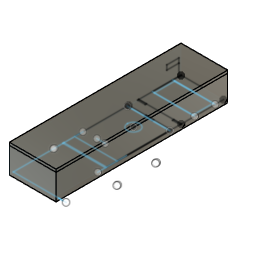
remotecase (Autodesk Fusion 360 design; units mm, degrees)
Autodesk Fusion 360 part; units mm, degrees
sketch "Sketch1" plane through (0, 0, 0) normal (0, 0, 1) x (1, 0, 0)
  line L0 (0, 0) -> (31, 0)
  line L1 (31, 0) -> (31, 114)
  line L2 (31, 114) -> (0, 114)
  line L3 (0, 114) -> (0, 0)
  dimension "d1" = 31
  dimension "d2" = 114
  constraint horizontal L0
  constraint vertical L1
  constraint horizontal L2
  constraint vertical L3
  constraint coincident L0.start L3.end
  measures "d1" distance of L0.start L0.end
  measures "d2" distance of L0.start L2.end
extrude "Extrude1" add sketch "Sketch1" along normal blind 9 makes body 1
sketch "Sketch2" plane through (0, 0, 9) normal (0, 0, 1) x (-1, 0, 0)
  line L0 (0, -114) -> (0, 0)
  line L1 (0, 0) -> (-31, 0)
  line L2 (-31, 0) -> (-31, -114)
  line L3 (-31, -114) -> (0, -114)
  line L4 (0, 0) -> (-1.4, 0)
  line L5 (-1.4, 0) -> (-1.4, -1.4)
  line L6 (-31, -114) -> (-29.6, -114)
  line L7 (-29.6, -114) -> (-29.6, -112.6)
  line L8 (-1.4, -1.4) -> (-29.6, -1.4)
  line L9 (-29.6, -1.4) -> (-29.6, -112.6)
  line L10 (-29.6, -112.6) -> (-1.4, -112.6)
  line L11 (-1.4, -112.6) -> (-1.4, -1.4)
  dimension "d5" = 1.4
  dimension "d6" = 1.4
  dimension "d7" = 1.4
  dimension "d8" = 1.4
  constraint coincident L0.end L1.start
  constraint perpendicular L0 L4
  constraint perpendicular L1 L5
  constraint coincident L2.end L3.start
  constraint perpendicular L2 L6
  constraint perpendicular L6 L7
  constraint horizontal L8
  constraint vertical L9
  constraint horizontal L10
  constraint vertical L11
  measures "d5" distance of L0.end L4.end
  measures "d6" distance of L4.end L5.end
  measures "d7" distance of L2.end L6.end
  measures "d8" distance of L6.end L7.end
extrude "Extrude2" cut sketch "Sketch2" against normal blind 7.2 contours L8 L9 L10 L11 bodies 1
sketch "Sketch3" plane through (0, 0, 1.8) normal (0, 0, 1) x (-1, 0, 0)
  line L0 (-1.4, -112.6) -> (-1.4, -1.4)
  line L1 (-1.4, -1.4) -> (-29.6, -1.4)
  line L2 (-29.6, -1.4) -> (-29.6, -112.6)
  line L3 (-29.6, -112.6) -> (-1.4, -112.6)
  line L4 (-29.6, -76.9421) -> (-29.6, -48.1421)
  line L5 (-15.5, -48.1421) -> (-10, -48.1421)
  line L6 (-1.4, -76.9421) -> (-29.6, -76.9421)
  line L7 (-15.5, -112.6) -> (-1.5, -112.6)
  line L8 (-1.5, -107.1) -> (-1.5, -112.6)
  line L9 (-1.5, -93.6) -> (-1.5, -107.1)
  line L10 (-29.6, -48.1421) -> (-29.6, -29.1421)
  line L11 (-43.6, -54.1421) -> (-43.6, -53.4421)
  line L12 (-1.4, -28.4421) -> (-1.4, -47.4421)
  line L13 (-43.6, -28.4421) -> (-43.6, -27.7421)
  line L14 (-36.4, -1.2421) -> (-1.4, -1.2421)
  line L15 (-1.4, -1.2421) -> (-1.4, -27.7421)
  line L16 (-15.5, -76.9421) -> (-15.5, -66.9421)
  circle A0 centre (-15.5, -66.9421) radius 4
  line L17 (-29.6, -76.9421) -> (-29.6, -41.9421)
  line L18 (-29.6, -41.9421) -> (-1.4, -41.9421)
  line L19 (-1.4, -41.9421) -> (-1.4, -76.9421)
  line L20 (-1.4, -76.9421) -> (-29.6, -76.9421)
  line L21 (-29.6, -76.9421) -> (-29.6, -41.9421)
  line L22 (-29.6, -41.9421) -> (-29.6, -34.9421)
  line L23 (-29.6, -34.9421) -> (-1.4, -34.9421)
  line L24 (-1.4, -34.9421) -> (-1.4, -34.2421)
  line L25 (-1.4, -34.2421) -> (-29.6, -34.2421)
  line L26 (-29.6, -34.2421) -> (-29.6, -34.9421)
  line L27 (-1.5, -107.1) -> (-29.5, -107.1074)
  line L28 (-1.5, -93.6) -> (-29.5, -93.5275)
  line L29 (-15.5, -107.1037) -> (-2.75, -107.1003)
  line L30 (-2.75, -107.1003) -> (-28.25, -107.1003)
  line L31 (-28.25, -107.1003) -> (-28.25, -93.5638)
  line L32 (-28.25, -93.5638) -> (-2.75, -93.5638)
  line L33 (-2.75, -93.5638) -> (-2.75, -107.1003)
  line L34 (-1.4, -112.6) -> (-1.4, -84.6)
  line L35 (-1.4, -84.6) -> (-6.4, -84.6)
  line L36 (-6.4, -84.6) -> (-6.4, -83.8)
  line L37 (-6.4, -83.8) -> (-1.4, -83.8)
  line L38 (-1.4, -83.8) -> (-1.4, -84.6)
  line L39 (-1.4, -84.6) -> (-29.6, -84.6)
  line L40 (-29.6, -84.6) -> (-24.6, -84.6)
  line L41 (-24.6, -84.6) -> (-24.6, -83.8)
  line L42 (-24.6, -83.8) -> (-29.6, -83.8)
  line L43 (-29.6, -83.8) -> (-29.6, -84.6)
  line L44 (-29.6, -112.6) -> (-29.6, -77.8)
  line L45 (-29.6, -77.8) -> (-1.4, -77.8)
  line L46 (-15.5, -77.8) -> (-13, -77.8)
  line L47 (-13, -77.8) -> (-18, -77.8)
  line L48 (-18, -77.8) -> (-18, -77)
  line L49 (-18, -77) -> (-13, -77)
  line L50 (-13, -77) -> (-13, -77.8)
  dimension "d23" = 14
  dimension "d25" = 5.5
  dimension "d26" = 13.5
  dimension "d53" = 10
  dimension "d54" = 8
  dimension "d58" = 35
  dimension "d59" = 7
  dimension "d60" = 0.7
  dimension "d61" = 12.75
  dimension "d62" = 25.5
  dimension "d122" = 28
  dimension "d123" = 5
  dimension "d124" = 0.8
  dimension "d125" = 5
  dimension "d126" = 0.8
  dimension "d131" = 34.8
  dimension "d132" = 2.5
  dimension "d133" = 5
  dimension "d134" = 0.8
  constraint coincident L2 L4.start
  constraint parallel L2 L4
  constraint perpendicular L0 L5
  constraint coincident L0 L6.start
  constraint perpendicular L4 L6
  constraint midpoint L3 L7.start
  constraint perpendicular L0 L7
  constraint vertical L8
  constraint vertical L9
  constraint vertical L11
  constraint vertical L12
  constraint vertical L13
  constraint horizontal L14
  constraint vertical L15
  constraint midpoint L6 L16.start
  constraint perpendicular L6 L16
  constraint coincident L16.end A0.centre
  constraint perpendicular L6 L17
  constraint horizontal L18
  constraint vertical L19
  constraint horizontal L20
  constraint vertical L21
  constraint perpendicular L18 L22
  constraint horizontal L23
  constraint vertical L24
  constraint horizontal L25
  constraint vertical L26
  constraint midpoint L27 L29.start
  constraint parallel L27 L29
  constraint horizontal L30
  constraint vertical L31
  constraint horizontal L32
  constraint vertical L33
  constraint coincident L0.start L3.end
  constraint perpendicular L3 L34
  constraint horizontal L35
  constraint vertical L36
  constraint horizontal L37
  constraint vertical L38
  constraint horizontal L39
  constraint coincident L2 L39.end
  constraint horizontal L40
  constraint vertical L41
  constraint horizontal L42
  constraint vertical L43
  constraint coincident L2.end L3.start
  constraint perpendicular L32 L44
  constraint coincident L0 L45.end
  constraint perpendicular L0 L45
  constraint midpoint L45 L46.start
  constraint parallel L45 L46
  constraint horizontal L47
  constraint vertical L48
  constraint horizontal L49
  constraint vertical L50
  measures "d23" distance of L7.start L7.end
  measures "d25" distance of L7.end L8.start
  measures "d26" distance of L8.start L9.start
  measures "d53" distance of L16.start L16.end
  measures "d54" diameter of A0
  measures "d58" distance of L4.start L17.end
  measures "d59" distance of L17.end L22.end
  measures "d60" distance of L22.end L25.end
  measures "d61" distance of L29.start L29.end
  measures "d62" distance of L29.end L30.end
  measures "d122" distance of L0.start L34.end
  measures "d123" distance of L34.end L35.end
  measures "d124" distance of L34.end L37.end
  measures "d125" distance of L39.end L40.end
  measures "d126" distance of L39.end L42.end
  measures "d131" distance of L2.end L44.end
  measures "d132" distance of L46.start L46.end
  measures "d133" distance of L46.end L47.end
  measures "d134" distance of L46.end L49.end
extrude "Extrude10" cut sketch "Sketch3" against normal blind 6 contours L28 L30 L31 L32 L33 bodies 1
extrude "Extrude11" cut sketch "Sketch3" against normal blind 6 contours A0 bodies 1
extrude "Extrude12" add 1 faces at (30.5333, 38.4667, 9) along direction (0, 0, 1) blind 8 on bodies 1 bodies 1
sketch "Sketch8" plane through (0, 114, 0) normal (0, 1, 0) x (-1, 0, 0)
  line L0 (-31, 0) -> (0, 0)
  line L1 (0, 0) -> (0, 17)
  line L2 (0, 17) -> (-31, 17)
  line L3 (-31, 17) -> (-31, 0)
  line L4 (-15.5, 0) -> (-15.5, 8)
  line L5 (-15.5, 8) -> (-27.5, 8)
  line L6 (-27.5, 8) -> (-27.5, 15)
  line L7 (-27.5, 15) -> (-15.5, 15)
  line L8 (-15.5, 15) -> (-15.5, 8)
  dimension "d74" = 8
  dimension "d75" = 12
  dimension "d76" = 7
  constraint midpoint L0 L4.start
  constraint perpendicular L0 L4
  constraint horizontal L5
  constraint vertical L6
  constraint horizontal L7
  constraint vertical L8
  measures "d74" distance of L4.start L4.end
  measures "d75" distance of L4.end L5.end
  measures "d76" distance of L4.end L7.end
extrude "Extrude14" cut sketch "Sketch8" against normal blind 18 contours L5 L6 L7 L8 bodies 1
sketch "Sketch3 (2)" plane through (0, 0, 17) normal (0, 0, 1) x (-1, 0, 0) in component "kapak"
  line L0 (-29.6, -1.4) -> (-1.4, -1.4)
  line L1 (-1.4, -1.4) -> (-1.4, -112.6)
  line L2 (-1.4, -112.6) -> (-29.6, -112.6)
  line L3 (-29.6, -112.6) -> (-29.6, -1.4)
  line L4 (0, -114) -> (0, 0)
  line L5 (0, 0) -> (-31, 0)
  line L6 (-31, 0) -> (-31, -114)
  line L7 (-31, -114) -> (0, -114)
  line L8 (0, -114) -> (-31, -114)
  line L9 (-31, -114) -> (-31, 0)
  line L10 (-31, 0) -> (0, 0)
  line L11 (0, 0) -> (0, -114)
  constraint horizontal L8
  constraint vertical L9
  constraint horizontal L10
  constraint vertical L11
  constraint coincident L5.end L6.start
  constraint coincident L4.start L7.end
extrude "Extrude1'" add sketch "Sketch3 (2)" along normal blind 1.8 separate body contours L0 L1 L2 L3 | L4 L5 L6 L7 L8 L9 L10 L11 makes body 2 in component "kapak"
sketch "Sketch4" plane through (0, 0, 17) normal (0, 0, 1) x (1, 0, 0) in component "kapak"
  line L0 (1.4, 1.4) -> (29.6, 1.4)
  line L1 (29.6, 1.4) -> (29.6, 112.6)
  line L2 (29.6, 112.6) -> (1.4, 112.6)
  line L3 (1.4, 112.6) -> (1.4, 1.4)
  line L4 (1.4, 1.4) -> (2.8, 1.4)
  line L5 (1.4, 2.8) -> (1.4, 1.4)
  line L6 (29.6, 112.6) -> (28.2, 112.6)
  line L7 (29.6, 111.2) -> (29.6, 112.6)
  line L8 (28.2, 111.2) -> (2.8, 111.2)
  line L9 (2.8, 111.2) -> (2.8, 2.8)
  line L10 (2.8, 2.8) -> (28.2, 2.8)
  line L11 (28.2, 2.8) -> (28.2, 111.2)
  dimension "d90" = 1.4
  dimension "d91" = 1.4
  dimension "d92" = 1.4
  dimension "d93" = 1.4
  constraint horizontal L0
  constraint vertical L1
  constraint horizontal L2
  constraint vertical L3
  constraint horizontal L4
  constraint vertical L5
  constraint horizontal L8
  constraint vertical L9
  constraint horizontal L10
  constraint vertical L11
  measures "d90" distance of L0.start L4.end
  measures "d91" distance of L0.start L5.start
  measures "d92" distance of L1.end L6.end
  measures "d93" distance of L1.end L7.start
extrude "Extrude2'" add sketch "Sketch4" against normal blind 1.2 bodies 2 in component "kapak"
sketch "Sketch6" plane through (0, 0, 17) normal (0, 0, -1) x (1, 0, 0) in component "kapak"
  line L0 (31, 0) -> (0, 0)
  line L1 (0, 0) -> (0, -114)
  line L2 (0, -114) -> (31, -114)
  line L3 (31, -114) -> (31, 0)
  line L4 (29.6, -112.6) -> (1.4, -112.6)
  line L5 (1.4, -112.6) -> (1.4, -1.4)
  line L6 (1.4, -1.4) -> (29.6, -1.4)
  line L7 (29.6, -1.4) -> (29.6, -112.6)
  line L8 (15.5, -114) -> (15.5, -104)
  line L9 (15.5, -104) -> (15.1, -104)
  line L10 (15.1, -104) -> (15.9, -104)
  line L11 (15.9, -104) -> (15.9, -89)
  line L12 (15.9, -89) -> (15.1, -89)
  line L13 (15.1, -89) -> (15.1, -104)
  line L14 (15.5, -114) -> (15.5, -64)
  line L15 (15.5, -64) -> (15.1, -64)
  line L16 (15.1, -64) -> (16.5, -64)
  line L17 (16.5, -64) -> (16.5, -54)
  line L18 (16.5, -54) -> (15.1, -54)
  line L19 (15.1, -54) -> (15.1, -64)
  line L20 (15.5, 0) -> (15.5, -10)
  line L21 (15.5, -10) -> (15.1, -10)
  line L22 (15.1, -10) -> (15.9, -10)
  line L23 (15.9, -10) -> (15.9, -20)
  line L24 (15.9, -20) -> (15.1, -20)
  line L25 (15.1, -20) -> (15.1, -10)
  dimension "d96" = 10
  dimension "d97" = 0.4
  dimension "d98" = 0.8
  dimension "d99" = 15
  dimension "d100" = 50
  dimension "d101" = 0.4
  dimension "d102" = 1.4
  dimension "d103" = 10
  dimension "d104" = 10
  dimension "d105" = 0.4
  dimension "d106" = 0.8
  dimension "d107" = 10
  constraint midpoint L2 L8.start
  constraint perpendicular L2 L8
  constraint perpendicular L8 L9
  constraint horizontal L10
  constraint vertical L11
  constraint horizontal L12
  constraint vertical L13
  constraint vertical L14
  constraint perpendicular L14 L15
  constraint horizontal L16
  constraint vertical L17
  constraint horizontal L18
  constraint vertical L19
  constraint midpoint L0 L20.start
  constraint perpendicular L6 L20
  constraint perpendicular L20 L21
  constraint horizontal L22
  constraint vertical L23
  constraint horizontal L24
  constraint vertical L25
  measures "d96" distance of L8.start L8.end
  measures "d97" distance of L8.end L9.end
  measures "d98" distance of L9.end L10.end
  measures "d99" distance of L9.end L12.end
  measures "d100" distance of L8.start L14.end
  measures "d101" distance of L14.end L15.end
  measures "d102" distance of L15.end L16.end
  measures "d103" distance of L15.end L18.end
  measures "d104" distance of L20.start L20.end
  measures "d105" distance of L20.end L21.end
  measures "d106" distance of L21.end L22.end
  measures "d107" distance of L21.end L24.end
extrude "Extrude3" add sketch "Sketch6" along normal blind 7.5 contours L21 L22 L23 L24 L25 bodies 2 in component "kapak"
extrude "Extrude4" add sketch "Sketch6" along normal blind 8 contours L15 L16 L17 L18 L19 bodies 2 in component "kapak"
extrude "Extrude5" add sketch "Sketch6" along normal blind 3.5 contours L10 L11 L12 L14 | L9 L10 L12 L13 L14 bodies 2 in component "kapak"
extrude "Extrude6" add 1 faces at (16.0333, 60.6667, 9) along direction (0, 0, -1) blind 2 on bodies 2 bodies 2 in component "kapak"
sketch "Sketch9" plane through (0, 0, 0) normal (-1, 0, 0) x (0, -1, 0)
  line L0 (-114, 0) -> (0, 0)
  line L1 (0, 0) -> (0, 17)
  line L2 (0, 17) -> (-114, 17)
  line L3 (-114, 17) -> (-114, 0)
  line L4 (-114, 0) -> (-112.6, 0)
  line L5 (-112.6, 0) -> (-112.6, 8)
  line L6 (-112.6, 8) -> (-104.6, 8)
  line L7 (-104.6, 8) -> (-104.6, 11)
  line L8 (-104.6, 11) -> (-112.6, 11)
  line L9 (-112.6, 11) -> (-112.6, 8)
  dimension "d116" = 1.4
  dimension "d117" = 8
  dimension "d118" = 8
  dimension "d119" = 3
  constraint coincident L0.start L3.end
  constraint perpendicular L3 L4
  constraint perpendicular L0 L5
  constraint horizontal L6
  constraint vertical L7
  constraint horizontal L8
  constraint vertical L9
  measures "d116" distance of L0.start L4.end
  measures "d117" distance of L4.end L5.end
  measures "d118" distance of L5.end L6.end
  measures "d119" distance of L5.end L8.end
extrude "Extrude15" cut sketch "Sketch9" against normal blind 3 contours L6 L7 L8 L9 bodies 1
sketch "Sketch10" plane through (0, 0, 1.8) normal (0, 0, 1) x (1, 0, 0)
extrude "Extrude16" add sketch "Sketch3" along normal blind 4 contours L2 L39 L40 L41 L42 L43 L44 bodies 1
extrude "Extrude17" add sketch "Sketch3" along normal blind 4 contours L0 L35 L36 L37 L38 L39 bodies 1
extrude "Extrude18" add sketch "Sketch3" along normal blind 11 contours L45 L46 L47 L48 L49 L50 bodies 1
extrude "Extrude7" cut 1 faces at (16.0333, 60.6667, 7) along direction (0, 0, 1) blind 1 on bodies 2 bodies 2 in component "kapak"
extrude "Extrude3'" [suppressed]
extrude "Extrude4'" [suppressed]
extrude "Extrude5'" [suppressed]
extrude "Extrude6'" [suppressed]
sketch "Sketch4 (2)" plane through (0, 0, 0) normal (0, -1, 0) x (1, 0, 0)
  line L0 (0, 0) -> (45, 0)
  line L1 (45, 0) -> (45, 9)
  line L2 (45, 9) -> (0, 9)
  line L3 (0, 9) -> (0, 0)
  line L4 (0, 0) -> (1.4, 0)
  line L5 (1.4, 0) -> (1.4, 1.8)
  line L6 (1.4, 1.8) -> (6.4, 1.8)
  line L7 (6.4, 1.8) -> (6.4, 6.8)
  line L8 (6.4, 6.8) -> (1.4, 6.8)
  line L9 (1.4, 6.8) -> (1.4, 1.8)
  dimension "d41" = 1.4
  dimension "d42" = 1.8
  dimension "d43" = 5
  dimension "d44" = 5
  constraint coincident L0.start L3.end
  constraint perpendicular L3 L4
  constraint perpendicular L4 L5
  constraint horizontal L6
  constraint vertical L7
  constraint horizontal L8
  constraint vertical L9
  measures "d41" distance of L0.start L4.end
  measures "d42" distance of L4.end L5.end
  measures "d43" distance of L5.end L6.end
  measures "d44" distance of L5.end L8.end
extrude "Extrude7'" [suppressed]
sketch "Sketch5" plane through (0, 0, 0) normal (-1, 0, 0) x (0, -1, 0)
  line L0 (-114, 0) -> (0, 0)
  line L1 (0, 0) -> (0, 9)
  line L2 (0, 9) -> (-114, 9)
  line L3 (-114, 9) -> (-114, 0)
  line L4 (0, 0) -> (0, 1.8)
  line L5 (0, 1.8) -> (-7.4, 1.8)
  line L6 (-7.4, 1.8) -> (-27.4, 1.8)
  line L7 (-27.4, 1.8) -> (-27.4, 6.8)
  line L8 (-27.4, 6.8) -> (-7.4, 6.8)
  line L9 (-7.4, 6.8) -> (-7.4, 1.8)
  dimension "d47" = 1.8
  dimension "d48" = 7.4
  dimension "d49" = 20
  dimension "d50" = 5
  constraint coincident L0.end L1.start
  constraint perpendicular L0 L4
  constraint perpendicular L4 L5
  constraint horizontal L6
  constraint vertical L7
  constraint horizontal L8
  constraint vertical L9
  measures "d47" distance of L0.end L4.end
  measures "d48" distance of L4.end L5.end
  measures "d49" distance of L5.end L6.end
  measures "d50" distance of L5.end L8.end
extrude "Extrude8" [suppressed]
extrude "Extrude9" [suppressed]
component "kapak" placed x (1, 0, 0) y (0, 1, 0) z (0, 0, 1) at (0, 0, 0)
